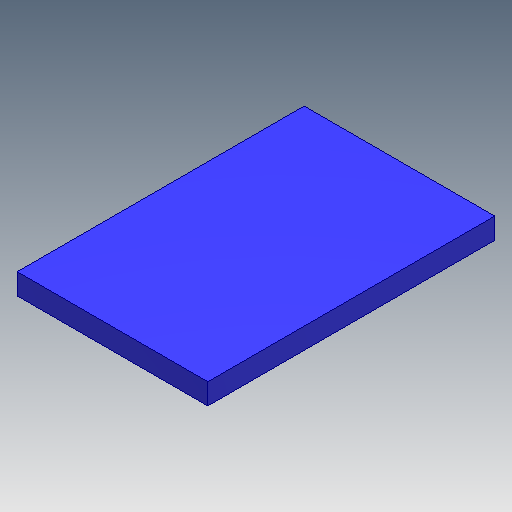
# Autodesk Inventor part: POWER_JACKPTH
Saved by Autodesk Inventor 2017 (Build 210142000, 142)
## iProperties
Part Number: POWER_JACKPTH
Material: Generisch
Document SubType Name: Modeling
Designer: Werkstatt
Density: 1 g/cm^3
Appearance: POWER_JACK_PTH, POWER_JACKPTH
Author: Werkstatt
Autodesk Inventor part; units mm, degrees
ref_plane "YZ Plane" through (0, 0, 0) normal (1, 0, 0) x (0, 1, 0)
ref_plane "XZ Plane" through (0, 0, 0) normal (0, 1, 0) x (-1, 0, 0)
ref_plane "XY Plane" through (0, 0, 0) normal (0, 0, 1) x (1, 0, 0)
sketch "POWER_JACK_PTH, POWER_JACKPTH_29" plane through (0, 0, 0) normal (0, 0, 1) x (1, 0, 0)
  line L0 (-4.5, 13.8016) -> (4.6016, 13.8016)
  line L1 (4.6016, 13.8016) -> (4.6016, 0.1)
  line L2 (4.6016, 0.1) -> (-4.5, 0.1)
  line L3 (-4.5, 0.1) -> (-4.5, 13.8016)
  constraints: 8 end point
extrude "Extrusion1" add sketch "POWER_JACK_PTH, POWER_JACKPTH_29" along normal blind 1
